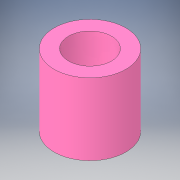
# Autodesk Inventor part: lozysko
Saved by Autodesk Inventor 2019 (Build 230136000, 136)
## iProperties
Created: 2020-01-12
Part Number: lozysko
Material: Ogólny
Document SubType Name: Modeling
Designer: Karolina
Density: 1 g/cm^3
Appearance: Domyślna
Author: Karolina
Autodesk Inventor part; units mm, degrees
ref_plane "YZ Plane" through (0, 0, 0) normal (1, 0, 0) x (0, 1, 0)
ref_plane "XZ Plane" through (0, 0, 0) normal (0, 1, 0) x (-1, 0, 0)
ref_plane "XY Plane" through (0, 0, 0) normal (0, 0, 1) x (1, 0, 0)
sketch "Szkic1" plane through (0, 0, 0) normal (0, 0, 1) x (1, 0, 0)
  line L0 (0.3, 0) -> (0.5, 0)
  line L1 (0.5, 0) -> (0.5, 1)
  line L2 (0.5, 1) -> (0.3, 1)
  line L3 (0.3, 1) -> (0.3, 0)
  line L4 (-0.1, 0) -> (0.6, 0) construction
  line L5 (0, -0.2) -> (0, 1.2) projected
  point P0 (0, 0)
  dimension "d0" = 0.3
  dimension "d1" = 0.5
  dimension "d2" = 1
  constraints: 8 end point, 2 parallel, 1 collinear, 1 horizontal, 1 perpendicular
  measures "d0" distance from line of point (0, 0) L3
  measures "d1" distance from line of point (0, 0) L1
  measures "d2" distance between parallel lines of L0 L2
revolve "Obrót1" add sketch "Szkic1" angle 360 about axis through (0, -10, 0) along (0, 1, 0)
